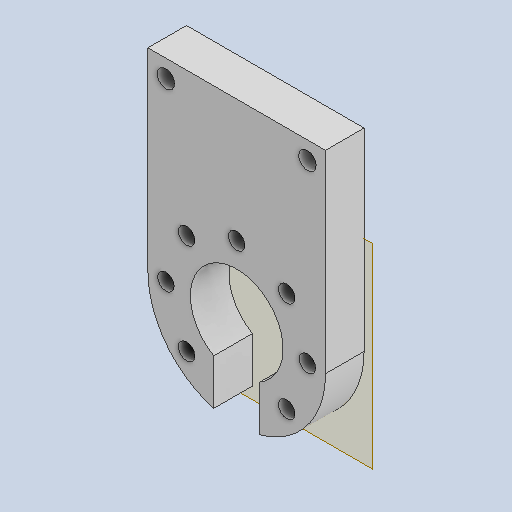
# Autodesk Inventor part: _thigh_2
Saved by Autodesk Inventor 2024.3 (Build 283343000, 343)
## iProperties
Created: 2024-09-06
Part Number: _thigh_2
Material: 일반
Document SubType Name: Modeling
Designer: gretc
Density: 1 g/cm^3
Appearance: 기본값
Author: gretc
Autodesk Inventor part; units mm, degrees
ref_plane "YZ Plane" through (0, 0, 0) normal (1, 0, 0) x (0, 1, 0)
ref_plane "XZ Plane" through (0, 0, 0) normal (0, 1, 0) x (-1, 0, 0)
ref_plane "XY Plane" through (0, 0, 0) normal (0, 0, 1) x (1, 0, 0)
ref_plane "작업 평면1" through (0, 0, 0) normal (0, 0, 1) x (1, 0, 0)
sketch "스케치1" plane through (0, 0, 0) normal (0, 0, 1) x (1, 0, 0)
  line L0 (3.5511, -14.2422) -> (3.5511, 14.2422) projected
  line L1 (-3.5511, 14.2422) -> (-3.5511, -14.2422) projected
  line L2 (-3.5511, -14.2422) -> (3.5511, -14.2422) projected
  circle A0 centre (0, 0) radius 13.8 projected
  line L3 (3.5511, 14.2422) -> (-3.5511, 14.2422) projected
  line L4 (13.8, 0) -> (13.8, 30.0667) projected
  line L5 (13.8, 30.0667) -> (-13.8, 30.0667) projected
  line L6 (-13.8, 30.0667) -> (-13.8, 0) projected
  circle A1 centre (0, 0) radius 13.8 projected
  circle A2 centre (0, 0) radius 7.2 projected
  circle A3 centre (0, -11) radius 1.2812 projected
  circle A4 centre (-7.7782, -7.7782) radius 1.2812 projected
  circle A5 centre (-11, 0) radius 1.2812 projected
  circle A6 centre (-7.7782, 7.7782) radius 1.2812 projected
  circle A7 centre (0, 11) radius 1.2812 projected
  circle A8 centre (7.7782, 7.7782) radius 1.2812 projected
  circle A9 centre (11, 0) radius 1.2812 projected
  circle A10 centre (7.7782, -7.7782) radius 1.2812 projected
  circle A11 centre (11, 27.3) radius 1.35 projected
  circle A12 centre (-11, 27.3) radius 1.35 projected
  point P0 (0, 0)
  point P1 (3.5511, -6.2634)
  point P2 (3.5511, -13.3353)
  point P3 (-3.5511, -13.3353)
  point P4 (-3.5511, -6.2634)
extrude "돌출1" add sketch "스케치1" along normal blind 6 contours L0 A2 A0 | A0 L1 A2 | A0 L0 L3 L1 L6 L5 L4 | A2 L1 A0 L0 | A0 L1 L3 L0 picked at (-2.7821, 10.0973)
